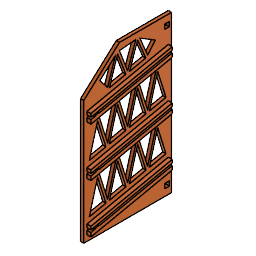
side-panel-left (Autodesk Fusion 360 design; units mm, degrees)
part number: 2026-08-18-20-59-32-920
Autodesk Fusion 360 part; units mm, degrees
sketch "Sketch1" plane through (0, 0, 0) normal (1, 0, 0) x (0, 0, -1)
  line L0 (0, 15) -> (0, 150)
  line L1 (0, 150) -> (-240, 150)
  line L2 (-240, 150) -> (-240, 70)
  line L3 (-240, 70) -> (-190, 15)
  line L4 (-190, 15) -> (0, 15)
extrude "Extrude1" add sketch "Sketch1" along normal blind 5 from surface at 3 makes body 1
sketch "Sketch2" plane through (0, 0, 0) normal (1, 0, 0) x (0, 0, -1)
  line L0 (-9, 20) -> (-35.5696, 145)
  line L1 (-35.5696, 145) -> (-41.5696, 145)
  line L2 (-41.5696, 145) -> (-15, 20)
  line L3 (-15, 20) -> (-9, 20)
extrude "Extrude2" add sketch "Sketch2" along normal blind 6 from surface at 8 separate body makes body 2
sketch "Sketch3" plane through (0, 0, 0) normal (1, 0, 0) x (0, 0, -1)
  line L0 (-18.2, 20) -> (-44.7696, 145)
  line L1 (-44.7696, 145) -> (-49.7696, 145)
  line L2 (-49.7696, 145) -> (-23.2, 20)
  line L3 (-23.2, 20) -> (-18.2, 20)
extrude "Extrude3" add sketch "Sketch3" along normal blind 6 from surface at 8 separate body makes body 3
sketch "Sketch4" plane through (0, 0, 0) normal (1, 0, 0) x (0, 0, -1)
  line L0 (-16.2753, 26) -> (-17.2753, 28)
  line L1 (-17.2753, 28) -> (-18.3381, 31)
  line L2 (-18.3381, 31) -> (-17.7632, 33)
  line L3 (-17.7632, 33) -> (-16.2753, 26)
extrude "Extrude4" add sketch "Sketch4" along normal blind 6 from surface at 8 separate body makes body 4
sketch "Sketch5" plane through (0, 0, 0) normal (1, 0, 0) x (0, 0, -1)
  line L0 (-84, 20) -> (-110.5696, 145)
  line L1 (-110.5696, 145) -> (-116.5696, 145)
  line L2 (-116.5696, 145) -> (-90, 20)
  line L3 (-90, 20) -> (-84, 20)
extrude "Extrude5" add sketch "Sketch5" along normal blind 6 from surface at 8 separate body makes body 5
sketch "Sketch6" plane through (0, 0, 0) normal (1, 0, 0) x (0, 0, -1)
  line L0 (-93.2, 20) -> (-119.7696, 145)
  line L1 (-119.7696, 145) -> (-124.7696, 145)
  line L2 (-124.7696, 145) -> (-98.2, 20)
  line L3 (-98.2, 20) -> (-93.2, 20)
extrude "Extrude6" add sketch "Sketch6" along normal blind 6 from surface at 8 separate body makes body 6
sketch "Sketch7" plane through (0, 0, 0) normal (1, 0, 0) x (0, 0, -1)
  line L0 (-91.2753, 26) -> (-92.2753, 28)
  line L1 (-92.2753, 28) -> (-93.3381, 31)
  line L2 (-93.3381, 31) -> (-92.7632, 33)
  line L3 (-92.7632, 33) -> (-91.2753, 26)
extrude "Extrude7" add sketch "Sketch7" along normal blind 6 from surface at 8 separate body makes body 7
sketch "Sketch8" plane through (0, 0, 0) normal (1, 0, 0) x (0, 0, -1)
  line L0 (-159, 20) -> (-185.5696, 145)
  line L1 (-185.5696, 145) -> (-191.5696, 145)
  line L2 (-191.5696, 145) -> (-165, 20)
  line L3 (-165, 20) -> (-159, 20)
extrude "Extrude8" add sketch "Sketch8" along normal blind 6 from surface at 8 separate body makes body 8
sketch "Sketch9" plane through (0, 0, 0) normal (1, 0, 0) x (0, 0, -1)
  line L0 (-168.2, 20) -> (-194.7696, 145)
  line L1 (-194.7696, 145) -> (-199.7696, 145)
  line L2 (-199.7696, 145) -> (-173.2, 20)
  line L3 (-173.2, 20) -> (-168.2, 20)
extrude "Extrude9" add sketch "Sketch9" along normal blind 6 from surface at 8 separate body makes body 9
sketch "Sketch10" plane through (0, 0, 0) normal (1, 0, 0) x (0, 0, -1)
  line L0 (-166.2753, 26) -> (-167.2753, 28)
  line L1 (-167.2753, 28) -> (-168.3381, 31)
  line L2 (-168.3381, 31) -> (-167.7632, 33)
  line L3 (-167.7632, 33) -> (-166.2753, 26)
extrude "Extrude10" add sketch "Sketch10" along normal blind 6 from surface at 8 separate body makes body 10
combine "Combine1" operation add target body 1 tool bodies 2 3 4 5 6 7 8 9 10
sketch "Sketch11" plane through (0, 0, 0) normal (1, 0, 0) x (0, 0, -1)
  line L0 (-10.5, 139.5) -> (-10.5, 146.5)
  line L1 (-10.5, 146.5) -> (-17.5, 146.5)
  line L2 (-17.5, 146.5) -> (-17.5, 139.5)
  line L3 (-17.5, 139.5) -> (-10.5, 139.5)
extrude "Extrude11" cut sketch "Sketch11" along normal blind 30 from surface at -2 bodies 1
sketch "Sketch12" plane through (0, 0, 0) normal (1, 0, 0) x (0, 0, -1)
  line L0 (-222.5, 139.5) -> (-222.5, 146.5)
  line L1 (-222.5, 146.5) -> (-229.5, 146.5)
  line L2 (-229.5, 146.5) -> (-229.5, 139.5)
  line L3 (-229.5, 139.5) -> (-222.5, 139.5)
extrude "Extrude12" cut sketch "Sketch12" along normal blind 30 from surface at -2 bodies 1
sketch "Sketch13" plane through (0, 0, 0) normal (1, 0, 0) x (0, 0, -1)
  line L0 (-31.0484, 23.6788) -> (-36.4457, 49.0712)
  line L1 (-36.4457, 49.0712) -> (-77.3478, 36.375)
  line L2 (-77.3478, 36.375) -> (-31.0484, 23.6788)
  line L3 (-37.5845, 54.4288) -> (-42.9818, 79.8212)
  line L4 (-42.9818, 79.8212) -> (-83.8839, 67.125)
  line L5 (-83.8839, 67.125) -> (-37.5845, 54.4288)
  line L6 (-44.1206, 85.1788) -> (-49.5179, 110.5712)
  line L7 (-49.5179, 110.5712) -> (-90.42, 97.875)
  line L8 (-90.42, 97.875) -> (-44.1206, 85.1788)
  line L9 (-50.6567, 115.9288) -> (-56.054, 141.3212)
  line L10 (-56.054, 141.3212) -> (-96.9561, 128.625)
  line L11 (-96.9561, 128.625) -> (-50.6567, 115.9288)
  line L12 (-80.9836, 39.0538) -> (-86.3809, 64.4462)
  line L13 (-86.3809, 64.4462) -> (-40.0815, 51.75)
  line L14 (-40.0815, 51.75) -> (-80.9836, 39.0538)
  line L15 (-87.5197, 69.8038) -> (-92.917, 95.1962)
  line L16 (-92.917, 95.1962) -> (-46.6176, 82.5)
  line L17 (-46.6176, 82.5) -> (-87.5197, 69.8038)
  line L18 (-94.0558, 100.5538) -> (-99.4532, 125.9462)
  line L19 (-99.4532, 125.9462) -> (-53.1537, 113.25)
  line L20 (-53.1537, 113.25) -> (-94.0558, 100.5538)
  line L21 (-106.0484, 23.6788) -> (-111.4457, 49.0712)
  line L22 (-111.4457, 49.0712) -> (-152.3478, 36.375)
  line L23 (-152.3478, 36.375) -> (-106.0484, 23.6788)
  line L24 (-112.5845, 54.4288) -> (-117.9818, 79.8212)
  line L25 (-117.9818, 79.8212) -> (-158.8839, 67.125)
  line L26 (-158.8839, 67.125) -> (-112.5845, 54.4288)
  line L27 (-119.1206, 85.1788) -> (-124.5179, 110.5712)
  line L28 (-124.5179, 110.5712) -> (-165.42, 97.875)
  line L29 (-165.42, 97.875) -> (-119.1206, 85.1788)
  line L30 (-125.6567, 115.9288) -> (-131.054, 141.3212)
  line L31 (-131.054, 141.3212) -> (-171.9561, 128.625)
  line L32 (-171.9561, 128.625) -> (-125.6567, 115.9288)
  line L33 (-155.9836, 39.0538) -> (-161.3809, 64.4462)
  line L34 (-161.3809, 64.4462) -> (-115.0815, 51.75)
  line L35 (-115.0815, 51.75) -> (-155.9836, 39.0538)
  line L36 (-162.5197, 69.8038) -> (-167.917, 95.1962)
  line L37 (-167.917, 95.1962) -> (-121.6176, 82.5)
  line L38 (-121.6176, 82.5) -> (-162.5197, 69.8038)
  line L39 (-169.0558, 100.5538) -> (-174.4532, 125.9462)
  line L40 (-174.4532, 125.9462) -> (-128.1537, 113.25)
  line L41 (-128.1537, 113.25) -> (-169.0558, 100.5538)
  line L42 (-187.2601, 54.5801) -> (-192.5931, 79.6699)
  line L43 (-192.5931, 79.6699) -> (-225.962, 67.125)
  line L44 (-225.962, 67.125) -> (-187.2601, 54.5801)
  line L45 (-193.6564, 85.4229) -> (-198.95, 110.3271)
  line L46 (-198.95, 110.3271) -> (-228.8992, 97.875)
  line L47 (-228.8992, 97.875) -> (-193.6564, 85.4229)
  line L48 (-204.0679, 39.8492) -> (-225.7036, 63.6508)
  line L49 (-225.7036, 63.6508) -> (-188.9887, 51.75)
  line L50 (-188.9887, 51.75) -> (-204.0679, 39.8492)
  line L51 (-229.0083, 69.9849) -> (-231.1396, 95.0151)
  line L52 (-231.1396, 95.0151) -> (-195.7186, 82.5)
  line L53 (-195.7186, 82.5) -> (-229.0083, 69.9849)
  line L54 (-229.6635, 101.4803) -> (-215.5016, 125.0197)
  line L55 (-215.5016, 125.0197) -> (-201.3558, 113.25)
  line L56 (-201.3558, 113.25) -> (-229.6635, 101.4803)
extrude "Extrude13" cut sketch "Sketch13" along normal blind 9 from surface at 1 bodies 1
named bodies: "Тело"
